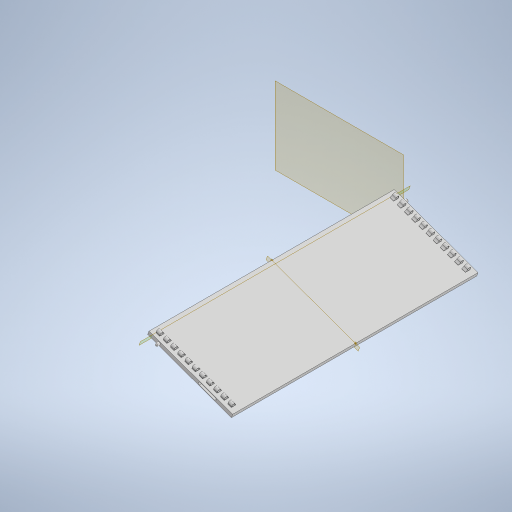
# Autodesk Inventor part: bed-base
Saved by Autodesk Inventor 2023 (Build 270158030, 158C)
## iProperties
Created: 2024-09-10
Part Number: bed-base
Material: Generic
Document SubType Name: Modeling
Designer: Imogen Heard
Density: 1 g/cm^3
Appearance: Default
Author: Imogen Heard
Autodesk Inventor part; units mm, degrees
ref_plane "YZ Plane" through (0, 0, 0) normal (1, 0, 0) x (0, 1, 0)
ref_plane "XZ Plane" through (0, 0, 0) normal (0, 1, 0) x (-1, 0, 0)
ref_plane "XY Plane" through (0, 0, 0) normal (0, 0, 1) x (1, 0, 0)
ref_plane "Work Plane4" through (0, 0, -7.700067) normal (0, 0, 1) x (1, 0, 0)
sketch "Sketch3" plane through (0, 0, -7.700067) normal (0, 0, 1) x (1, 0, 0)
  line L0 (623.930188, -108.857192) -> (189.330256, 47.399564)
  line L1 (623.930188, -108.857192) -> (576.737597, -506.063511)
  line L2 (576.737597, -506.063511) -> (646.248703, -514.322214)
  line L3 (646.248703, -514.322214) -> (683.53893, -200.461213)
  line L4 (683.53893, -200.461213) -> (983.972341, -468.849759)
  line L5 (983.972341, -468.849759) -> (978.073267, -518.500549)
  line L6 (978.073267, -518.500549) -> (1047.584373, -526.759252)
  line L7 (1047.584373, -526.759252) -> (1092.417334, -149.413249)
  line L8 (1092.417334, -149.413249) -> (1022.906228, -141.154546)
  line L9 (1022.906228, -141.154546) -> (994.054356, -383.992367)
  line L10 (994.054356, -383.992367) -> (693.620945, -115.603822)
  line L11 (693.620945, -115.603822) -> (699.340367, -67.465106)
  line L12 (699.340367, -67.465106) -> (635.486255, -59.878517)
  line L13 (206.247135, 94.450805) -> (635.486255, -59.878517)
  line L14 (201.510409, 81.276457) -> (206.247135, 94.450805)
  arc A0 (646.051866, -176.942663) -> (657.161838, -168.19232) centre (647.231681, -167.012505) ccw
  line L15 (636.121708, -175.762849) -> (646.051866, -176.942663)
  arc A1 (627.371365, -164.652876) -> (636.121708, -175.762849) centre (637.301523, -165.832691) ccw
  line L16 (632.090624, -124.932244) -> (627.371365, -164.652876)
  arc A2 (643.200596, -116.181901) -> (632.090624, -124.932244) centre (642.020782, -126.112059) ccw
  line L17 (653.130754, -117.361716) -> (643.200596, -116.181901)
  arc A3 (661.881098, -128.471688) -> (653.130754, -117.361716) centre (651.95094, -127.291874) ccw
  line L18 (657.161838, -168.19232) -> (661.881098, -128.471688)
  arc A4 (615.376682, -435.12677) -> (626.486655, -426.376427) centre (616.556497, -425.196612) ccw
  line L19 (605.446524, -433.946956) -> (615.376682, -435.12677)
  arc A5 (596.696181, -422.836983) -> (605.446524, -433.946956) centre (606.626339, -424.016798) ccw
  line L20 (601.41544, -383.116351) -> (596.696181, -422.836983)
  arc A6 (612.525412, -374.366008) -> (601.41544, -383.116351) centre (611.345598, -384.296166) ccw
  line L21 (622.45557, -375.545823) -> (612.525412, -374.366008)
  arc A7 (631.205914, -386.655795) -> (622.45557, -375.545823) centre (621.275756, -385.475981) ccw
  line L22 (626.486655, -426.376427) -> (631.205914, -386.655795)
  arc A8 (623.045478, -370.580744) -> (634.155451, -361.8304) centre (624.225293, -360.650586) ccw
  line L23 (613.11532, -369.400929) -> (623.045478, -370.580744)
  arc A9 (604.364977, -358.290956) -> (613.11532, -369.400929) centre (614.295135, -359.470771) ccw
  line L24 (609.084236, -318.570324) -> (604.364977, -358.290956)
  arc A10 (620.194208, -309.819981) -> (609.084236, -318.570324) centre (619.014394, -319.750139) ccw
  line L25 (630.124366, -310.999796) -> (620.194208, -309.819981)
  arc A11 (638.87471, -322.109769) -> (630.124366, -310.999796) centre (628.944552, -320.929954) ccw
  line L26 (634.155451, -361.8304) -> (638.87471, -322.109769)
  arc A12 (638.38307, -241.48869) -> (649.493042, -232.738347) centre (639.562885, -231.558532) ccw
  line L27 (628.452912, -240.308875) -> (638.38307, -241.48869)
  arc A13 (619.702569, -229.198903) -> (628.452912, -240.308875) centre (629.632727, -230.378717) ccw
  line L28 (624.421828, -189.478271) -> (619.702569, -229.198903)
  arc A14 (635.5318, -180.727928) -> (624.421828, -189.478271) centre (634.351986, -190.658086) ccw
  line L29 (645.461958, -181.907742) -> (635.5318, -180.727928)
  arc A15 (654.212302, -193.017715) -> (645.461958, -181.907742) centre (644.282144, -191.8379) ccw
  line L30 (649.493042, -232.738347) -> (654.212302, -193.017715)
  arc A16 (607.707886, -499.672797) -> (618.817859, -490.922454) centre (608.887701, -489.742639) ccw
  line L31 (597.777728, -498.492982) -> (607.707886, -499.672797)
  arc A17 (589.027385, -487.38301) -> (597.777728, -498.492982) centre (598.957543, -488.562824) ccw
  line L32 (593.746644, -447.662378) -> (589.027385, -487.38301)
  arc A18 (604.856617, -438.912035) -> (593.746644, -447.662378) centre (603.676802, -448.842193) ccw
  line L33 (614.786774, -440.091849) -> (604.856617, -438.912035)
  arc A19 (623.537118, -451.201822) -> (614.786774, -440.091849) centre (613.60696, -450.022007) ccw
  line L34 (618.817859, -490.922454) -> (623.537118, -451.201822)
  arc A20 (630.714274, -306.034717) -> (641.824247, -297.284374) centre (631.894089, -296.104559) ccw
  line L35 (620.784116, -304.854902) -> (630.714274, -306.034717)
  arc A21 (612.033773, -293.744929) -> (620.784116, -304.854902) centre (621.963931, -294.924744) ccw
  line L36 (616.753032, -254.024298) -> (612.033773, -293.744929)
  arc A22 (627.863004, -245.273954) -> (616.753032, -254.024298) centre (626.68319, -255.204112) ccw
  line L37 (637.793162, -246.453769) -> (627.863004, -245.273954)
  arc A23 (646.543506, -257.563742) -> (637.793162, -246.453769) centre (636.613348, -256.383927) ccw
  line L38 (641.824247, -297.284374) -> (646.543506, -257.563742)
  line L39 (197.418756, 55.118125) -> (207.568883, 83.348869)
  line L40 (207.568883, 83.348869) -> (866.286249, -153.48743)
  line L41 (866.286249, -153.48743) -> (856.136121, -181.718174)
  line L42 (856.136121, -181.718174) -> (197.418756, 55.118125)
  line L43 (194.066982, 60.573912) -> (288.169463, 26.740155)
  line L44 (189.330256, 47.399564) -> (194.066982, 60.573912)
  line L45 (295.612889, 47.442701) -> (201.510409, 81.276457)
  arc A24 (288.169463, 26.740155) -> (295.612889, 47.442701) centre (291.891176, 37.091428) ccw
  point P0 (0, 0)
  dimension "d1" = 700
  dimension "d2" = 30
  dimension "d3" = 5
  dimension "d4" = 10
  constraints: 8 end point, 2 parallel, 2 perpendicular
  measures "d1" distance between parallel lines of L41 L39
  measures "d2" distance between parallel lines of L40 L42
  measures "d3" distance between parallel lines of L14 L39
  measures "d4" distance between parallel lines of L42 L0
sketch "Sketch3 outline for Extrusion1" plane through (0, 0, -7.700067) normal (0, 0, 1) x (1, 0, 0)
  line L0 (856.136121, -181.718174) -> (866.286249, -153.48743)
  line L1 (197.418756, 55.118125) -> (856.136121, -181.718174)
  line L2 (207.568883, 83.348869) -> (197.418756, 55.118125)
  line L3 (866.286249, -153.48743) -> (207.568883, 83.348869)
extrude "Extrusion1" add sketch "Sketch3 outline for Extrusion1" along normal blind 1930
sketch "Sketch4" plane through (0, 0, 1922.299933) normal (0, 0, 1) x (1, 0, 0)
  circle A0 centre (605.831287, -74.720432) radius 10
  line L0 (605.831287, -75.783103) -> (725.831287, -118.928096) construction
  line L1 (602.109574, -86.134376) -> (722.109574, -129.279369)
  line L2 (729.553, -108.576823) -> (609.553, -65.431831)
  arc A1 (609.553, -65.431831) -> (602.109574, -86.134376) centre (605.831287, -75.783103) ccw
  arc A2 (722.109574, -129.279369) -> (729.553, -108.576823) centre (725.831287, -118.928096) ccw
  line L3 (197.418756, 55.118125) -> (856.136121, -181.718174)
  line L4 (866.286249, -153.48743) -> (207.568883, 83.348869)
  line L5 (665.831287, -97.3556) -> (836.523068, -158.726397) construction
  point P0 (0, 0)
  point P1 (526.777439, -63.300025)
  point P2 (609.37928, -65.371007)
  point P3 (602.283294, -65.371007)
  dimension "d7" = 22
  dimension "d8" = 4
  dimension "d9" = 4
  dimension "d11" = 0
  dimension "d21" = 120
  constraints: 10 end point, 4 point on circle, 4 tangent, 2 centre point, 2 midpoint, 2 parallel, 1 point on line
  measures "d7" distance between parallel lines of L1 L2
  measures "d8" distance from line of point (526.777, -63.3) L1
  measures "d9" distance between parallel lines of L4 L2
  measures "d11" horizontal distance of L0.start A0.centre
  measures "d21" horizontal distance of L0.end A0.centre
sketch "Sketch4 outline for Extrusion2" plane through (0, 0, 1922.299933) normal (0, 0, 1) x (1, 0, 0)
  line L0 (729.553, -108.576823) -> (609.553, -65.431831)
  arc A0 (609.553, -65.431831) -> (609.37928, -65.371007) centre (605.831287, -75.783103) ccw
  arc A1 (609.37928, -65.371007) -> (602.109574, -86.134376) centre (605.831287, -75.783103) ccw
  line L1 (602.109574, -86.134376) -> (722.109574, -129.279369)
  arc A2 (722.109574, -129.279369) -> (729.553, -108.576823) centre (725.831287, -118.928096) ccw
extrude "Extrusion2" cut sketch "Sketch4 outline for Extrusion2" against normal blind 30
sketch "Sketch5" plane through (0, 0, 1922.299933) normal (0, 0, 1) x (1, 0, 0)
  circle A0 centre (287.186052, 38.783115) radius 10
  line L0 (197.418756, 55.118125) -> (856.136121, -181.718174)
  line L1 (866.286249, -153.48743) -> (207.568883, 83.348869)
  line L2 (207.568883, 83.348869) -> (197.418756, 55.118125)
  point P0 (0, 0)
  dimension "d14" = 20
  dimension "d15" = 15
  dimension "d16" = 15
  dimension "d17" = 90
  constraints: 1 centre point
  measures "d14" diameter of A0
  measures "d15" distance from line of L0 A0.centre
  measures "d16" distance from line of L1 A0.centre
  measures "d17" distance from line of L2 A0.centre
sketch "Sketch5 outline for Extrusion3" plane through (0, 0, 1922.299933) normal (0, 0, 1) x (1, 0, 0)
  circle A0 centre (287.186052, 38.783115) radius 10
extrude "Extrusion3" add sketch "Sketch5 outline for Extrusion3" along normal blind 25 separate body
fillet "Fillet1" radius 6 1 edges at (277.1861, 38.7831, 1947.2999)
ref_plane "Work Plane5" through (225.6495, 44.967998, -7.700067) normal (-0.9410248, 0.3383376, 0) x (0, 0, 1)
sketch "Sketch6" plane through (225.6495, 44.967998, -7.700067) normal (-0.9410248, 0.3383376, 0) x (0, 0, 1)
  circle A0 centre (1892.5, 44) radius 10
  circle A1 centre (1892.5, 44) radius 12.5
  line L0 (0, 30) -> (1930, 30)
  line L1 (1903.5, 30) -> (1867.5, 30)
  line L2 (1867.5, 30) -> (1867.5, 33)
  line L3 (1867.5, 33) -> (1903.5, 33)
  line L4 (1903.5, 33) -> (1903.5, 30)
  arc A2 (1867.5, 33) -> (1880.365339, 47) centre (1860.976437, 51.906166) ccw
  arc A3 (1902.856158, 37) -> (1903.5, 33) centre (1908.753996, 35.897503) ccw
  point P0 (7.700067, -118.661705)
  point P1 (1867.5, 30)
  dimension "d23" = 2.5
  dimension "d24" = 11
  dimension "d25" = 25
  dimension "d26" = 3
  dimension "d27" = 4
  dimension "d28" = 6
  dimension "d29" = 3
  dimension "d30" = 20
  constraints: 8 end point, 6 point on circle, 3 centre point, 2 parallel, 1 horizontal, 1 perpendicular, 1 point on line
  measures "d23" radial gap between concentric circles of A1 A0
  measures "d24" distance from line of A0.centre L4
  measures "d25" distance from line of A0.centre L2
  measures "d26" vertical distance of A0.centre A1.start
  measures "d27" distance from line of L3 A1.end
  measures "d28" radius of A3
  measures "d29" distance between parallel lines of L3 L0
  measures "d30" radius of A2
sketch "Sketch6 outline for Extrusion4" plane through (225.6495, 44.967998, -7.700067) normal (-0.9410248, 0.3383376, 0) x (0, 0, 1)
  arc A0 (1880.365339, 47) -> (1867.5, 33) centre (1860.976437, 51.906166) cw
  arc A1 (1902.856158, 37) -> (1880.365339, 47) centre (1892.5, 44) ccw
  line L0 (1867.5, 33) -> (1867.5, 30)
  arc A2 (1903.5, 33) -> (1902.856158, 37) centre (1908.753996, 35.897503) cw
  line L1 (1867.5, 30) -> (1903.5, 30)
  line L2 (1903.5, 30) -> (1903.5, 33)
  circle A3 centre (1892.5, 44) radius 10
extrude "Extrusion4" add sketch "Sketch6 outline for Extrusion4" against normal blind 30 separate body
pattern_linear "Rectangular Pattern1" count 11 spacing 60 along (0.9410248, -0.3383376, 0) of "Extrusion4" bodies 3
ref_plane "Work Plane6" through (207.568883, 83.348869, 957.299933) normal (0, 0, 1) x (-0.3383376, -0.9410248, 0)
mirror "Mirror1" about plane through (207.568883, 83.348869, 957.299933) normal (0, 0, 1) of "Extrusion4", "Rectangular Pattern1" bodies 1
mirror "Mirror2" about plane through (207.568883, 83.348869, 957.299933) normal (0, 0, 1) of "Extrusion2", "Fillet1", "Extrusion3" bodies 1
